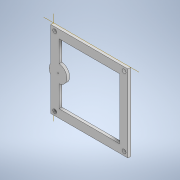
# Autodesk Inventor part: P2
Saved by Autodesk Inventor 2022 (Build 260153000, 153)
## iProperties
Created: 2022-11-21
Part Number: P2
Material: Genérico
Document SubType Name: Modeling
Designer: javie
Density: 1 g/cm^3
Appearance: Valor por defecto
Autodesk Inventor part; units mm, degrees
ref_plane "YZ Plane" through (0, 0, 0) normal (1, 0, 0) x (0, 1, 0)
ref_plane "XZ Plane" through (0, 0, 0) normal (0, 1, 0) x (-1, 0, 0)
ref_plane "XY Plane" through (0, 0, 0) normal (0, 0, 1) x (1, 0, 0)
sketch "Boceto1" plane through (0, 0, 0) normal (0, 0, 1) x (1, 0, 0)
  circle A0 centre (812.7165, -188.8432) radius 3.5
  circle A1 centre (938.7165, -188.8432) radius 3.5
  circle A2 centre (812.7165, -314.8432) radius 3.5
  circle A3 centre (938.7165, -314.8432) radius 3.5
  circle A4 centre (7, -133) radius 3.5
  circle A5 centre (7, -7) radius 3.5
  circle A6 centre (133, -133) radius 3.5
  circle A7 centre (133, -7) radius 3.5
  circle A8 centre (742.932, -379.7007) radius 3.5
  circle A9 centre (684.4665, -289.064) radius 3.5
  line L0 (643.3746, -238.0566) -> (643.3746, -186.384)
  line L1 (643.3746, -186.384) -> (658.3746, -186.384)
  line L2 (658.3746, -186.384) -> (658.3746, -231.5095)
  circle A10 centre (650.6272, -198.084) radius 3.5
  line L3 (930.7165, -299.4631) -> (930.7165, -313.8432)
  line L4 (930.7165, -313.8432) -> (820.7165, -313.8432)
  line L5 (820.7165, -313.8432) -> (820.7165, -299.8432)
  line L6 (820.7165, -299.8432) -> (820.7165, -267.7177)
  arc A11 (802.6937, -413.4304) -> (798.6937, -413.4304) centre (800.6937, -413.4304) ccw
  line L7 (802.6937, -413.4304) -> (802.6937, -450.6101)
  arc A12 (798.6937, -450.6101) -> (802.6937, -450.6101) centre (800.6937, -450.6101) ccw
  line L8 (798.6937, -450.6101) -> (798.6937, -413.4304)
  line L9 (899.1229, -399.4144) -> (899.1229, -391.9144)
  line L10 (899.1229, -391.9144) -> (815.1529, -391.9144)
  arc A13 (812.4407, -391.5396) -> (815.1529, -391.9144) centre (815.1529, -381.9144) ccw
  line L11 (812.4407, -391.5396) -> (788.253, -384.724)
  arc A14 (788.253, -384.724) -> (786.3475, -384.3818) centre (785.5409, -394.3492) ccw
  arc A15 (784.4303, -384.0363) -> (786.3475, -384.3818) centre (787.1541, -374.4144) ccw
  line L12 (718.1963, -348.8257) -> (755.3759, -348.8257)
  arc A16 (755.3759, -348.8257) -> (755.3759, -344.8257) centre (755.3759, -346.8257) ccw
  line L13 (755.3759, -344.8257) -> (718.1963, -344.8257)
  arc A17 (718.1963, -344.8257) -> (718.1963, -348.8257) centre (718.1963, -346.8257) ccw
  line L14 (0, -60.6726) -> (0, 0)
  line L15 (0, 0) -> (140, 0)
  line L16 (140, 0) -> (140, -140)
  line L17 (140, -140) -> (0, -140)
  line L18 (0, -140) -> (0, -79.3274)
  line L19 (15, -85.8745) -> (15, -125)
  line L20 (15, -125) -> (125, -125)
  line L21 (125, -125) -> (125, -15)
  line L22 (125, -15) -> (15, -15)
  line L23 (15, -15) -> (15, -54.1255)
  line L24 (-993.9843, 33.9517) -> (-715.1465, 33.9517)
  line L25 (-715.1465, 33.9517) -> (-715.1465, -156.5278)
  line L26 (-715.1465, -156.5278) -> (-993.9843, -156.5278)
  line L27 (-993.9843, -156.5278) -> (-993.9843, 33.9517)
  circle A18 centre (-961.4218, 1.0641) radius 2.5
  circle A19 centre (-835.4218, 1.0641) radius 2.5
  circle A20 centre (-961.4218, -124.9359) radius 2.5
  circle A21 centre (-835.4218, -124.9359) radius 2.5
  line L28 (-1001.1961, 41.4488) -> (-685.1452, 41.4488)
  line L29 (-685.1452, 41.4488) -> (-685.1452, -163.7638)
  line L30 (-685.1452, -163.7638) -> (-1001.1961, -163.7638)
  line L31 (-1001.1961, -163.7638) -> (-1001.1961, 41.4488)
  circle A22 centre (938.6116, -461.4421) radius 3.5
  line L32 (832.2485, -453.4421) -> (930.6116, -453.4421)
  line L33 (930.6116, -453.4421) -> (930.6116, -414.3166)
  line L34 (832.2485, -468.4421) -> (832.2485, -453.4421)
  line L35 (832.2485, -328.4421) -> (945.6116, -328.4421)
  line L36 (945.6116, -328.4421) -> (945.6116, -389.1147)
  line L37 (832.2485, -343.4421) -> (832.2485, -328.4421)
  circle A23 centre (938.6116, -335.4421) radius 3.5
  circle A24 centre (-821.7113, -229.9218) radius 8.1
  circle A25 centre (-864.2113, -229.9218) radius 3.25
  circle A26 centre (-839.0318, -229.9218) radius 3.25
  circle A27 centre (-932.7072, -191.2961) radius 3.25
  circle A28 centre (-915.3867, -191.2961) radius 8.1
  circle A29 centre (-957.8867, -191.2961) radius 3.25
  circle A30 centre (-864.0658, -191.0106) radius 3.25
  circle A31 centre (-838.8863, -191.0106) radius 3.25
  circle A32 centre (-821.5658, -191.0106) radius 8.1
  circle A33 centre (-881.7113, -229.9218) radius 7
  circle A34 centre (-974.6846, -229.7987) radius 7
  circle A35 centre (-957.1846, -229.7987) radius 3.25
  circle A36 centre (-932.0051, -229.7987) radius 3.25
  circle A37 centre (-914.6846, -229.7987) radius 8.1
  line L38 (-993.2367, -169.6143) -> (-798.5871, -169.6143)
  line L39 (-798.5871, -169.6143) -> (-798.5871, -253.6689)
  line L40 (-798.5871, -253.6689) -> (-993.2367, -253.6689)
  line L41 (-993.2367, -253.6689) -> (-993.2367, -169.6143)
  arc A38 (-924.0111, -244.6064) -> (-932.0051, -242.2987) centre (-932.0051, -257.2987) ccw
  line L42 (-932.0051, -242.2987) -> (-974.6846, -242.2987)
  arc A39 (-974.6846, -217.2987) -> (-974.6846, -242.2987) centre (-974.6846, -229.7987) ccw
  line L43 (-974.6846, -217.2987) -> (-932.0051, -217.2987)
  arc A40 (-932.0051, -217.2987) -> (-924.0111, -214.991) centre (-932.0051, -202.2987) ccw
  arc A41 (-924.0111, -244.6064) -> (-924.0111, -214.991) centre (-914.6846, -229.7987) ccw
  arc A42 (-881.7113, -217.4218) -> (-881.7113, -242.4218) centre (-881.7113, -229.9218) ccw
  line L44 (-881.7113, -217.4218) -> (-839.0318, -217.4218)
  arc A43 (-839.0318, -217.4218) -> (-831.0377, -215.1141) centre (-839.0318, -202.4218) ccw
  arc A44 (-831.0377, -244.7295) -> (-831.0377, -215.1141) centre (-821.7113, -229.9218) ccw
  arc A45 (-831.0377, -244.7295) -> (-839.0318, -242.4218) centre (-839.0318, -257.4218) ccw
  line L45 (-839.0318, -242.4218) -> (-881.7113, -242.4218)
  line L46 (-966.6367, -196.3479) -> (-975.3867, -201.3997)
  line L47 (-975.3867, -201.3997) -> (-984.1367, -196.3479)
  line L48 (-984.1367, -196.3479) -> (-984.1367, -186.2443)
  line L49 (-984.1367, -186.2443) -> (-975.3867, -181.1925)
  line L50 (-975.3867, -181.1925) -> (-966.6367, -186.2443)
  line L51 (-966.6367, -186.2443) -> (-966.6367, -196.3479)
  arc A46 (-924.7131, -206.1038) -> (-924.7131, -176.4884) centre (-915.3867, -191.2961) ccw
  arc A47 (-932.7072, -178.7961) -> (-924.7131, -176.4884) centre (-932.7072, -163.7961) ccw
  line L52 (-932.7072, -178.7961) -> (-975.3867, -178.7961)
  arc A48 (-975.3867, -178.7961) -> (-975.3867, -203.7961) centre (-975.3867, -191.2961) ccw
  line L53 (-975.3867, -203.7961) -> (-932.7072, -203.7961)
  arc A49 (-924.7131, -206.1038) -> (-932.7072, -203.7961) centre (-932.7072, -218.7961) ccw
  line L54 (-881.5658, -203.5106) -> (-838.8863, -203.5106)
  arc A50 (-830.8922, -205.8183) -> (-838.8863, -203.5106) centre (-838.8863, -218.5106) ccw
  arc A51 (-830.8922, -205.8183) -> (-830.8922, -176.2029) centre (-821.5658, -191.0106) ccw
  arc A52 (-838.8863, -178.5106) -> (-830.8922, -176.2029) centre (-838.8863, -163.5106) ccw
  line L55 (-838.8863, -178.5106) -> (-881.5658, -178.5106)
  arc A53 (-881.5658, -178.5106) -> (-881.5658, -203.5106) centre (-881.5658, -191.0106) ccw
  line L56 (-890.3158, -185.9588) -> (-881.5658, -180.907)
  line L57 (-881.5658, -180.907) -> (-872.8158, -185.9588)
  line L58 (-872.8158, -185.9588) -> (-872.8158, -196.0624)
  line L59 (-872.8158, -196.0624) -> (-881.5658, -201.1142)
  line L60 (-881.5658, -201.1142) -> (-890.3158, -196.0624)
  line L61 (-890.3158, -196.0624) -> (-890.3158, -185.9588)
  arc A54 (0, -60.6726) -> (0, -79.3274) centre (13, -70) ccw
  arc A55 (643.3746, -238.0566) -> (643.3746, -256.7114) centre (656.3746, -247.384) ccw
  arc A56 (805.7165, -242.5158) -> (805.7165, -261.1706) centre (818.7165, -251.8432) ccw
  arc A57 (679.4665, -307.4948) -> (688.8022, -330.5623) centre (693.4587, -315.2549) ccw
  arc A58 (930.6116, -382.5675) -> (930.6116, -414.3166) centre (932.6116, -398.4421) ccw
  arc A59 (753.3527, -391.3948) -> (780.9993, -399.4144) centre (769.1229, -388.6929) ccw
  arc A60 (15, -85.8745) -> (15, -54.1255) centre (13, -70) ccw
  line L62 (679.4665, -307.4948) -> (679.4665, -282.064)
  line L63 (679.4665, -282.064) -> (694.4606, -282.064)
  line L64 (694.4606, -282.064) -> (694.4606, -293.9069)
  arc A61 (694.4606, -293.9069) -> (696.1607, -299.4847) centre (704.4606, -293.9069) ccw
  line L65 (704.1803, -327.1313) -> (704.1803, -331.9041)
  arc A62 (704.1803, -331.9041) -> (704.5551, -334.6163) centre (714.1803, -331.9041) ccw
  line L66 (704.5551, -334.6163) -> (706.8683, -342.8257)
  line L67 (706.8683, -342.8257) -> (758.8683, -342.8257)
  arc A63 (758.8683, -350.8257) -> (758.8683, -342.8257) centre (759.1244, -346.8257) ccw
  line L68 (758.8683, -350.8257) -> (709.1225, -350.8257)
  line L69 (709.1225, -350.8257) -> (711.3055, -358.5727)
  arc A64 (711.6803, -361.2849) -> (711.3055, -358.5727) centre (701.6803, -361.2849) ccw
  line L70 (711.6803, -361.2849) -> (711.6803, -445.2549)
  line L71 (711.6803, -445.2549) -> (696.6803, -445.2549)
  line L72 (696.6803, -445.2549) -> (696.6803, -361.2849)
  arc A65 (696.6803, -361.2849) -> (696.3055, -358.5727) centre (686.6803, -361.2849) ccw
  line L73 (696.3055, -358.5727) -> (689.4899, -334.385)
  arc A66 (689.1477, -332.4795) -> (689.4899, -334.385) centre (699.1151, -331.6729) ccw
  arc A67 (689.1477, -332.4795) -> (688.8022, -330.5623) centre (679.1803, -333.2861) ccw
  arc A68 (704.1803, -327.1313) -> (696.1607, -299.4847) centre (693.4587, -315.2549) ccw
  line L74 (820.7165, -235.9687) -> (820.7165, -189.8432)
  line L75 (820.7165, -189.8432) -> (930.7165, -189.8432)
  line L76 (930.7165, -189.8432) -> (930.7165, -243.3432)
  line L77 (930.7165, -243.3432) -> (945.7165, -243.3432)
  line L78 (945.7165, -243.3432) -> (945.7165, -181.8432)
  line L79 (945.7165, -181.8432) -> (805.7165, -181.8432)
  line L80 (805.7165, -181.8432) -> (805.7165, -242.5158)
  line L81 (805.7165, -261.1706) -> (805.7165, -321.8432)
  line L82 (805.7165, -321.8432) -> (945.7165, -321.8432)
  line L83 (945.7165, -321.8432) -> (945.7165, -260.3432)
  line L84 (945.7165, -260.3432) -> (930.7165, -260.3432)
  line L85 (930.7165, -260.3432) -> (930.7165, -299.8432)
  arc A69 (820.7165, -267.7177) -> (820.7165, -235.9687) centre (818.7165, -251.8432) ccw
  line L86 (670.5079, -239.884) -> (793.3746, -239.884)
  line L87 (793.3746, -239.884) -> (793.3746, -254.884)
  line L88 (793.3746, -254.884) -> (670.5079, -254.884)
  line L89 (658.3746, -263.2585) -> (658.3746, -308.384)
  line L90 (658.3746, -308.384) -> (643.3746, -308.384)
  line L91 (643.3746, -308.384) -> (643.3746, -256.7114)
  arc A70 (658.3746, -263.2585) -> (670.5079, -254.884) centre (656.3746, -247.384) ccw
  arc A71 (670.5079, -239.884) -> (658.3746, -231.5095) centre (656.3746, -247.384) ccw
  line L92 (945.6116, -407.7694) -> (945.6116, -468.4421)
  line L93 (945.6116, -468.4421) -> (832.2485, -468.4421)
  line L94 (930.6116, -382.5675) -> (930.6116, -343.4421)
  line L95 (930.6116, -343.4421) -> (832.2485, -343.4421)
  arc A72 (945.6116, -407.7694) -> (945.6116, -389.1147) centre (932.6116, -398.4421) ccw
  line L96 (780.9993, -399.4144) -> (785.7722, -399.4144)
  arc A73 (788.4843, -399.7892) -> (785.7722, -399.4144) centre (785.7722, -409.4144) ccw
  line L97 (788.4843, -399.7892) -> (796.6937, -402.1024)
  line L98 (796.6937, -402.1024) -> (796.6937, -454.1024)
  arc A74 (796.6937, -454.1024) -> (804.6937, -454.1024) centre (800.6937, -454.3585) ccw
  line L99 (804.6937, -454.1024) -> (804.6937, -404.3566)
  line L100 (804.6937, -404.3566) -> (812.4407, -406.5396)
  arc A75 (812.4407, -406.5396) -> (815.1529, -406.9144) centre (815.1529, -396.9144) ccw
  line L101 (815.1529, -406.9144) -> (899.1229, -406.9144)
  line L102 (899.1229, -406.9144) -> (899.1229, -391.9144)
  line L103 (761.3628, -374.7007) -> (735.932, -374.7007)
  line L104 (735.932, -374.7007) -> (735.932, -389.6948)
  line L105 (735.932, -389.6948) -> (747.775, -389.6948)
  arc A76 (753.3527, -391.3948) -> (747.775, -389.6948) centre (747.775, -399.6948) ccw
  arc A77 (784.4303, -384.0363) -> (761.3628, -374.7007) centre (769.1229, -388.6929) ccw
  line L106 (930.7165, -243.3432) -> (930.7165, -260.3432)
  line L107 (945.7165, -243.3432) -> (945.7165, -260.3432)
  line L108 (628.631, -19.6698) -> (960.631, -19.6698)
  line L109 (960.631, -19.6698) -> (960.631, -482.6698)
  line L110 (960.631, -482.6698) -> (628.631, -482.6698)
  line L111 (628.631, -482.6698) -> (628.631, -19.6698)
  circle A78 centre (13, -70) radius 1
  point P0 (0, -463)
  point P1 (332, -463)
  point P2 (332, 0)
  point P3 (50.8356, -262.3941)
  point P4 (65.8296, -262.3941)
  point P5 (65.8296, -274.2371)
  point P6 (67.5297, -279.8148)
  point P7 (75.5493, -307.4614)
  point P8 (75.5493, -312.2343)
  point P9 (75.9241, -314.9465)
  point P10 (78.2373, -323.1558)
  point P11 (130.2373, -323.1558)
  point P12 (130.2373, -331.1558)
  point P13 (80.4915, -331.1558)
  point P14 (82.6745, -338.9029)
  point P15 (83.0493, -341.615)
  point P16 (83.0493, -425.585)
  point P17 (68.0493, -425.585)
  point P18 (68.0493, -341.615)
  point P19 (67.6745, -338.9029)
  point P20 (60.8589, -314.7152)
  point P21 (60.5167, -312.8096)
  point P22 (60.1712, -310.8924)
  point P23 (50.8356, -287.825)
  point P24 (316.9806, -388.0996)
  point P25 (316.9806, -448.7722)
  point P26 (203.6175, -448.7722)
  point P27 (203.6175, -433.7722)
  point P28 (301.9806, -433.7722)
  point P29 (301.9806, -394.6467)
  point P30 (301.9806, -362.8977)
  point P31 (301.9806, -323.7722)
  point P32 (203.6175, -323.7722)
  point P33 (203.6175, -308.7722)
  point P34 (316.9806, -308.7722)
  point P35 (316.9806, -369.4448)
  point P36 (15.3452, -75.2432)
  point P37 (15.3452, -14.5706)
  point P38 (155.3452, -14.5706)
  point P39 (155.3452, -154.5706)
  point P40 (15.3452, -154.5706)
  point P41 (15.3452, -93.898)
  point P42 (178.1524, -75.2432)
  point P43 (178.1524, -14.5706)
  point P44 (318.1524, -14.5706)
  point P45 (318.1524, -154.5706)
  point P46 (178.1524, -154.5706)
  point P47 (178.1524, -93.898)
  point P48 (29.7436, -243.5887)
  point P49 (29.7436, -288.7142)
  point P50 (14.7436, -288.7142)
  point P51 (14.7436, -237.0415)
  point P52 (14.7436, -218.3868)
  point P53 (14.7436, -166.7142)
  point P54 (29.7436, -166.7142)
  point P55 (29.7436, -211.8397)
  point P56 (41.8769, -220.2142)
  point P57 (164.7436, -220.2142)
  point P58 (164.7436, -235.2142)
  point P59 (41.8769, -235.2142)
  point P60 (186.5219, -372.2445)
  point P61 (270.4919, -372.2445)
  point P62 (270.4919, -379.7445)
  point P63 (270.4919, -387.2445)
  point P64 (186.5219, -387.2445)
  point P65 (183.8098, -386.8697)
  point P66 (176.0627, -384.6868)
  point P67 (176.0627, -434.4326)
  point P68 (168.0627, -434.4326)
  point P69 (168.0627, -382.4326)
  point P70 (159.8533, -380.1194)
  point P71 (157.1412, -379.7445)
  point P72 (152.3683, -379.7445)
  point P73 (124.7217, -371.725)
  point P74 (119.144, -370.0249)
  point P75 (107.301, -370.0249)
  point P76 (107.301, -355.0308)
  point P77 (132.7318, -355.0308)
  point P78 (155.7993, -364.3664)
  point P79 (157.7165, -364.712)
  point P80 (159.622, -365.0542)
  point P81 (183.8098, -371.8697)
  point P82 (317.0855, -240.6733)
  point P83 (317.0855, -302.1733)
  point P84 (177.0855, -302.1733)
  point P85 (177.0855, -241.5007)
  point P86 (177.0855, -222.846)
  point P87 (177.0855, -162.1733)
  point P88 (317.0855, -162.1733)
  point P89 (317.0855, -223.6733)
  dimension "d10" = 316.0509
  dimension "d11" = 295.1177
  dimension "d12" = 2
  constraints: 224 end point, 94 point on circle, 79 centre point, 1 coincident
  measures "d10" distance of L28.start L28.end
  measures "d11" vertical distance of L29.start L39.end
  measures "d12" diameter of A78
extrude "Extrusión2" add sketch "Boceto1" along normal blind 5 contours L14 L15 L16 L17 L18 A54
